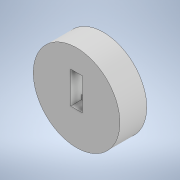
# Autodesk Inventor part: podstawa 01-4
Saved by Autodesk Inventor 2021 (Build 250183000, 183)
## iProperties
Created: 2022-02-04
Part Number: podstawa 01-4
Material: Generic
Document SubType Name: Modeling
Designer: Łukasz
Density: 1 g/cm^3
Appearance: Default
Author: Łukasz
Autodesk Inventor part; units mm, degrees
ref_plane "YZ Plane" through (0, 0, 0) normal (1, 0, 0) x (0, 1, 0)
ref_plane "XZ Plane" through (0, 0, 0) normal (0, 1, 0) x (-1, 0, 0)
ref_plane "XY Plane" through (0, 0, 0) normal (0, 0, 1) x (1, 0, 0)
sketch "Sketch1" plane through (0, 0, 0) normal (0, 0, 1) x (1, 0, 0)
  circle A0 centre (0, 0) radius 75
  dimension "d0" = 150
  constraints: 1 centre point, 1 coincident
  measures "d0" diameter of A0
extrude "Extrusion1" add sketch "Sketch1" along normal blind 46.5
sketch "Sketch2" plane through (0, 0, 46.5) normal (0, 0, 1) x (1, 0, 0)
  line L0 (-10.25, 30.375) -> (10.25, 30.375)
  line L1 (10.25, 30.375) -> (10.25, -10.125)
  line L2 (10.25, -10.125) -> (-10.25, -10.125)
  line L3 (-10.25, -10.125) -> (-10.25, 30.375)
  line L4 (3.25, -10.125) -> (-3.25, -10.125)
  line L5 (-3.25, -10.125) -> (-3.25, -15.125)
  line L6 (-3.25, -15.125) -> (3.25, -15.125)
  line L7 (3.25, -15.125) -> (3.25, -10.125)
  point P0 (0, 0)
  point P1 (-3.25, -10.125)
  dimension "d5" = 20.5
  dimension "d6" = 40.5
  dimension "d8" = 10.125
  dimension "d9" = 10.25
  dimension "d10" = 6.5
  dimension "d11" = 5
  dimension "d12" = 0
  dimension "d13" = 7
  constraints: 16 end point, 4 parallel, 2 horizontal, 2 perpendicular, 1 other
  measures "d5" distance of L1.end L2.end
  measures "d6" distance of L0.end L1.end
  measures "d8" distance from line of point (0, 0) L2
  measures "d9" distance from line of point (0, 0) L3
  measures "d10" distance of L6.end L5.end
  measures "d11" distance of L5.end L4.end
  measures "d12" distance between parallel lines of L2 L4
  measures "d13" distance between parallel lines of L3 L5
extrude "Extrusion2" cut sketch "Sketch2" against normal up to surface (46.5 mm away)
sketch "Sketch4" plane through (0, 0, 0) normal (0, 0, -1) x (-1, 0, 0)
  line L0 (2.5, -79.3047) -> (-2.5, -79.3047)
  line L1 (-2.5, -79.3047) -> (-2.5, -3.4585)
  line L2 (-2.5, -3.4585) -> (2.5, -3.4585)
  line L3 (2.5, -3.4585) -> (2.5, -79.3047)
  line L4 (-3.25, -15.125) -> (-3.25, -10.125) projected
  point P0 (0, 0)
  dimension "d16" = 5
  dimension "d17" = 0.75
  constraints: 8 end point, 2 parallel, 1 horizontal, 1 perpendicular
  measures "d16" distance of L1.end L2.end
  measures "d17" distance between parallel lines of L4 L1
extrude "Extrusion3" cut sketch "Sketch4" against normal blind 2.5
sketch "Sketch5" plane through (0, 0, 46.5) normal (0, 0, 1) x (1, 0, 0)
  line L0 (10.25, -17.625) -> (-10.25, -17.625)
  line L1 (-10.25, -17.625) -> (-10.25, 37.875)
  line L2 (-10.25, 37.875) -> (10.25, 37.875)
  line L3 (10.25, 37.875) -> (10.25, -17.625)
  line L4 (-10.25, 30.375) -> (10.25, 30.375) projected
  point P0 (0, 0)
  dimension "d20" = 55.5
  dimension "d21" = 7.5
  constraints: 8 end point, 2 parallel, 1 horizontal, 1 perpendicular
  measures "d20" distance of L0.end L1.end
  measures "d21" distance between parallel lines of L4 L2
extrude "Extrusion4" cut sketch "Sketch5" against normal blind 19
equation "\"d9\" = 0.5 * d5"
equation "\"d13\" = 0.5 * d5 - 0.5 * d10"
body "Solid1"
